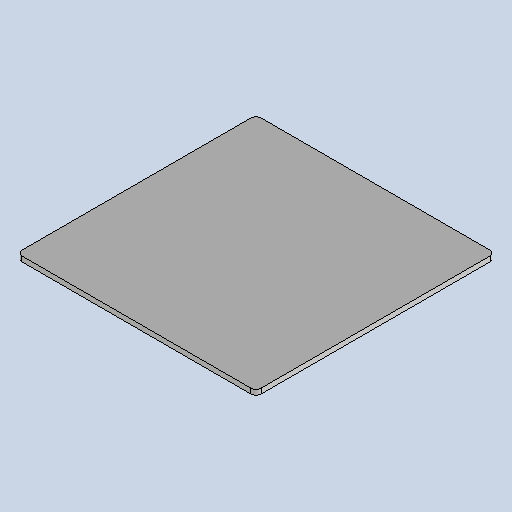
# Autodesk Inventor part: PNS 765 FDS 1200 CUP 1_1600
Saved by Autodesk Inventor 2025 (Build 290162010, 162A)
## iProperties
Created: 2025-06-24
Part Number: PNS 765 FDS 1200 CUP 1_1600
Material: Stainless Steel
Document SubType Name: Sheet Metal
Designer: admin
Mass: 141.321 g
Surface Area: 184.103 cm^2
Volume: 17.6651 cm^3
Density: 8 g/cm^3
Flat Pattern Width: 9.4 cm
Flat Pattern Length: 9.4 cm
Flat Pattern Area: 88.36 cm^2
Sheet Metal Rule: AISI304 2mm Die16
Sheet Metal Width: 94.000 mm
Sheet Metal Length: 94.000 mm
Sheet Metal Area: 8836.000 mm^2
Appearance: Default
Author: user
Autodesk Inventor part; units mm, degrees
ref_plane "YZ Plane" through (0, 0, 0) normal (1, 0, 0) x (0, 1, 0)
ref_plane "XZ Plane" through (0, 0, 0) normal (0, 1, 0) x (-1, 0, 0)
ref_plane "XY Plane" through (0, 0, 0) normal (0, 0, 1) x (1, 0, 0)
sketch "Sketch1" plane through (0, 0, 0) normal (0, 0, 1) x (1, 0, 0)
  line L0 (-47, -47) -> (47, -47)
  line L1 (47, -47) -> (47, 47)
  line L2 (47, 47) -> (-47, 47)
  line L3 (-47, 47) -> (-47, -47)
  line L4 (-47, -47) -> (47, 47) construction
  line L5 (47, -47) -> (-47, 47) construction
  point P0 (0, 0)
  dimension "d154" = 94
  dimension "d155" = 94
  measures "d154" distance of L1.end L2.end
  measures "d155" distance of L0.end L1.end
extrude "Plate5" add sketch "Sketch1" along normal blind 2
fillet "Corner Round1" radius 2 4 edges at (47, 47, 1) (-47, 47, 1) (-47, -47, 1) (47, -47, 1)
body "Solid3"
